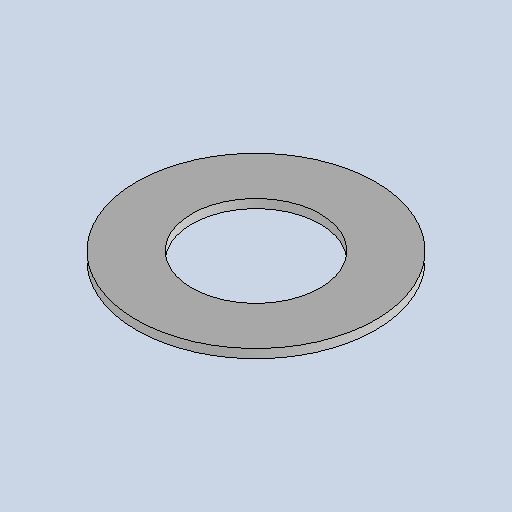
# Autodesk Inventor part: PNS 1792 FDS free flange DN50
Saved by Autodesk Inventor 2025.1 (Build 291241020, 241B)
## iProperties
Created: 2025-02-13
Part Number: PNS 1792 FDS free flange DN50
Material: Steel
Document SubType Name: Sheet Metal
Designer: user
Mass: 204.69 g
Surface Area: 151.236 cm^2
Volume: 26.0752 cm^3
Density: 7.85 g/cm^3
Flat Pattern Width: 10.8 cm
Flat Pattern Length: 10.8 cm
Flat Pattern Area: 116.64 cm^2
Sheet Metal Rule: AISI304 4mm Die 32
Sheet Metal Width: 108.000 mm
Sheet Metal Length: 108.000 mm
Sheet Metal Area: 11664.000 mm^2
Appearance: Default
Author: pokla
Autodesk Inventor part; units mm, degrees
ref_plane "YZ Plane" through (0, 0, 0) normal (1, 0, 0) x (0, 1, 0)
ref_plane "XZ Plane" through (0, 0, 0) normal (0, 1, 0) x (-1, 0, 0)
ref_plane "XY Plane" through (0, 0, 0) normal (0, 0, 1) x (1, 0, 0)
sketch "Sketch2" plane through (0, 0, 0) normal (0, 0, 1) x (1, 0, 0)
  circle A0 centre (0, 0) radius 29
  circle A1 centre (0, 0) radius 54
  dimension "d25" = 58
  dimension "d27" = 108
  measures "d25" diameter of A0
  measures "d27" diameter of A1
extrude "Plate2" add sketch "Sketch2" along normal blind 4
equation "\"d14\" = Thickness"
equation "\"BendReliefWidth\" = Thickness"
equation "\"BendReliefDepth\" = 0.5 * Thickness"
equation "\"CornerReliefSize\" = 4 * Thickness"
equation "\"MinimumRemnant\" = 2 * Thickness"
equation "\"TransitionRadius\" = BendRadius"
equation "\"JacobiRadiusSize\" = BendRadius"
equation "\"GapSize\" = Thickness"
equation "\"Thickness\" = 4"
equation "\"BendRadius\" = 6"
body "Solid3"
